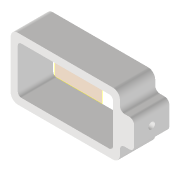
# Autodesk Inventor part: Holisheet_NEMA8_connector
Saved by Autodesk Inventor 2022 (Build 260153000, 153)
## iProperties
Created: 2023-03-11
Part Number: Holisheet_NEMA8_connector
Material: Generisch
Document SubType Name: Modeling
Designer: diederichbenedict
Density: 1 g/cm^3
Appearance: Vorgabe
Author: diederichbenedict
Autodesk Inventor part; units mm, degrees
ref_plane "YZ Plane" through (0, 0, 0) normal (1, 0, 0) x (0, 1, 0)
ref_plane "XZ Plane" through (0, 0, 0) normal (0, 1, 0) x (-1, 0, 0)
ref_plane "Arbeitsebene1" through (0, 0, -15) normal (0, 0, 1) x (1, 0, 0)
sketch "Skizze1" plane through (0, 0, -15) normal (0, 0, 1) x (1, 0, 0)
  line L0 (29.6698, 8.5) -> (29.6698, -8.5)
  arc A0 (29.6698, 8.5) -> (28.1698, 10) centre (28.1698, 8.5) ccw
  line L1 (11.1698, 10) -> (28.1698, 10)
  arc A1 (11.1698, 10) -> (9.6698, 8.5) centre (11.1698, 8.5) ccw
  line L2 (9.6698, -8.5) -> (9.6698, 8.5)
  arc A2 (9.6698, -8.5) -> (11.1698, -10) centre (11.1698, -8.5) ccw
  line L3 (28.1698, -10) -> (11.1698, -10)
  arc A3 (28.1698, -10) -> (29.6698, -8.5) centre (28.1698, -8.5) ccw
  circle A4 centre (27.6698, 8) radius 0.7835
  circle A5 centre (27.6698, -8) radius 0.7835
  circle A6 centre (11.6698, 8) radius 0.7835
  circle A7 centre (11.6698, -8) radius 0.7835
  circle A8 centre (19.6698, 0) radius 7.5
  line L4 (4.2698, 10) -> (4.2698, 8.9) projected
  line L5 (-5.8302, 10) -> (4.2698, 10) projected
  line L6 (-5.8302, 8.5) -> (-5.8302, 10) projected
  arc A9 (-9.3302, 5) -> (-5.8302, 8.5) centre (-9.3302, 8.5) ccw projected
  line L7 (-10.8302, 5) -> (-9.3302, 5) projected
  line L8 (-10.8302, -5) -> (-10.8302, 5) projected
  line L9 (-9.3302, -5) -> (-10.8302, -5) projected
  arc A10 (-5.8302, -8.5) -> (-9.3302, -5) centre (-9.3302, -8.5) ccw projected
  line L10 (-5.8302, -10) -> (-5.8302, -8.5) projected
  line L11 (4.2698, -10) -> (-5.8302, -10) projected
  line L12 (4.2698, -8.9) -> (4.2698, -10) projected
  arc A11 (7.6698, -5.5) -> (4.2698, -8.9) centre (7.6698, -8.9) ccw projected
  line L13 (11.1698, -5.5) -> (7.6698, -5.5)
  line L14 (11.1698, -5) -> (11.1698, -5.5)
  line L15 (11.1698, -5) -> (7.3698, -5)
  line L16 (7.3698, -5) -> (7.3698, 5)
  line L17 (7.3698, 5) -> (11.1698, 5)
  line L18 (11.1698, 5.5) -> (11.1698, 5)
  line L19 (7.6698, 5.5) -> (11.1698, 5.5)
  arc A12 (4.2698, 8.9) -> (7.6698, 5.5) centre (7.6698, 8.9) ccw projected
  circle A13 centre (-0.8302, 0) radius 2 projected
  line L20 (9.1698, 8.5) -> (9.1698, -8.5)
  arc A14 (9.1698, 8.5) -> (7.6698, 10) centre (7.6698, 8.5) ccw
  line L21 (-9.3302, 10) -> (7.6698, 10)
  arc A15 (-9.3302, 10) -> (-10.8302, 8.5) centre (-9.3302, 8.5) ccw
  line L22 (-10.8302, -8.5) -> (-10.8302, 8.5)
  arc A16 (-10.8302, -8.5) -> (-9.3302, -10) centre (-9.3302, -8.5) ccw
  line L23 (7.6698, -10) -> (-9.3302, -10)
  arc A17 (7.6698, -10) -> (9.1698, -8.5) centre (7.6698, -8.5) ccw
  circle A18 centre (7.1698, 8) radius 0.7835
  circle A19 centre (7.1698, -8) radius 0.7835
  circle A20 centre (-8.8302, 8) radius 0.7835
  circle A21 centre (-8.8302, -8) radius 0.7835
  circle A22 centre (-0.8302, 0) radius 7.5
  line L24 (-9.3302, -5.5) -> (-12.8302, -5.5)
  line L25 (-9.3302, -5) -> (-9.3302, -5.5)
  line L26 (-9.3302, -5) -> (-13.1302, -5)
  line L27 (-13.1302, 5) -> (-9.3302, 5)
  line L28 (-9.3302, 5.5) -> (-9.3302, 5)
  line L29 (-12.8302, 5.5) -> (-9.3302, 5.5)
  line L30 (11.1698, 10) -> (7.6698, 10)
  line L31 (11.1698, -10) -> (7.6698, -10)
  line L32 (-10.858, 10.25) -> (29.642, 10.25)
  line L33 (29.642, 10.25) -> (29.642, -10.25)
  line L34 (29.642, -10.25) -> (-10.858, -10.25)
  line L35 (-10.858, -10.25) -> (-10.858, 10.25)
  line L36 (-10.858, 10.25) -> (29.642, -10.25) construction
  line L37 (29.642, 10.25) -> (-10.858, -10.25) construction
  line L38 (32.642, -10.25) -> (32.642, 10.25)
  line L39 (29.642, 13.25) -> (-10.858, 13.25)
  line L40 (-13.858, 10.25) -> (-13.858, -10.25)
  line L41 (-10.858, -13.25) -> (29.642, -13.25)
  arc A23 (32.642, 10.25) -> (29.642, 13.25) centre (29.642, 10.25) ccw
  arc A24 (29.642, -13.25) -> (32.642, -10.25) centre (29.642, -10.25) ccw
  arc A25 (-13.858, -10.25) -> (-10.858, -13.25) centre (-10.858, -10.25) ccw
  arc A26 (-10.858, 13.25) -> (-13.858, 10.25) centre (-10.858, 10.25) ccw
  line L42 (38.642, 6) -> (32.642, 6)
  line L43 (32.642, 6) -> (32.642, -6)
  line L44 (32.642, -6) -> (38.642, -6)
  line L45 (38.642, -6) -> (38.642, 6)
  line L46 (38.642, 6) -> (32.642, -6) construction
  line L47 (32.642, 6) -> (38.642, -6) construction
  point P0 (0, 0)
  point P1 (9.392, 0)
  point P2 (35.642, 0)
  point P3 (32.642, 0)
  point P4 (29.642, -8.7873)
  point P5 (29.642, 8.7873)
  dimension "d1" = 20.5
  dimension "d2" = 3
  dimension "d3" = 3
  dimension "d6" = 6
  dimension "d7" = 12
  constraints: 78 end point, 24 point on circle, 22 centre point, 8 tangent, 7 parallel, 6 midpoint, 3 equal radius, 3 horizontal, 3 perpendicular, 3 other
  measures "d1" distance of L32.end L33.end
  measures "d2" distance between parallel lines of L33 L38
  measures "d3" radius of A23
  measures "d6" distance of L44.end L43.end
  measures "d7" distance of L43.end L42.end
extrude "Extrusion1" add sketch "Skizze1" along normal blind 15 contours L0 A3 L33 A0 | A0 L1 L30 L21 L5 A15 L22 L29 L35 L32 L33 | L33 L34 L35 L24 L22 A16 L23 L11 L31 L3 A3 | L29 L22 L27 L35 | L35 L26 L22 L24 | L27 L8 L26 L35 | A24 L41 A25 L40 A26 L39 A23 L38 | L38 L42 L45 L44
fillet "Rundung1" radius 2 4 edges at (32.642, 6, -7.5) (38.642, 6, -7.5) (38.642, -6, -7.5) (32.642, -6, -7.5)
sketch "Skizze2" plane through (38.642, -4, -15) normal (1, 0, 0) x (0, 0, -1)
  line L0 (0, 0) -> (-15, 0) projected
  line L1 (0, 0) -> (0, 8) projected
  line L2 (-15, 8) -> (0, 8) projected
  line L3 (-15, 0) -> (-15, 8) projected
  circle A0 centre (-7.5, 4) radius 1.4
  point P0 (-15, 4)
  dimension "d9" = 2.8
  constraints: 1 centre point
  measures "d9" diameter of A0
extrude "Extrusion2" cut sketch "Skizze2" against normal blind 15 contours A0
